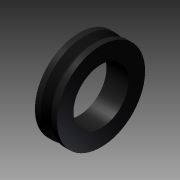
# Autodesk Inventor part: 8 ball cable roller
Saved by Autodesk Inventor 2012 (Build 160160000, 160)
## iProperties
Created: 2013-12-03
Part Number: 8 ball cable roller
Material: Default
Document SubType Name: Modeling
Designer: Bryce
Density: 1 g/cm^3
Author: Bryce
Autodesk Inventor part; units mm, degrees
ref_plane "YZ Plane" through (0, 0, 0) normal (1, 0, 0) x (0, 1, 0)
ref_plane "XZ Plane" through (0, 0, 0) normal (0, 1, 0) x (-1, 0, 0)
ref_plane "XY Plane" through (0, 0, 0) normal (0, 0, 1) x (1, 0, 0)
sketch "Sketch1" plane through (0, 0, 0) normal (0, 0, 1) x (1, 0, 0)
  line L0 (0, 0) -> (9.525, 0) construction
  line L1 (1.5875, 7.9375) -> (7.9375, 7.9375)
  line L2 (7.9375, 7.9375) -> (7.9375, 12.7)
  line L3 (1.5875, 12.7) -> (1.5875, 7.9375)
  line L4 (3.175, 12.7) -> (4.7625, 11.1125)
  line L5 (4.7625, 11.1125) -> (6.35, 12.7)
  line L6 (7.9375, 12.7) -> (6.35, 12.7)
  line L7 (3.175, 12.7) -> (1.5875, 12.7)
  line L8 (1.5875, 7.9375) -> (0, 7.9375)
  line L9 (0, 7.9375) -> (0, 6.6675)
  line L10 (0, 6.6675) -> (0.635, 6.6675)
  line L11 (0.635, 6.6675) -> (0.635, 5.08)
  line L12 (0.635, 5.08) -> (0, 5.08)
  line L13 (0, 5.08) -> (0, 2.54)
  line L14 (0, 2.54) -> (9.525, 2.54)
  line L15 (9.525, 2.54) -> (9.525, 5.08)
  line L16 (9.525, 5.08) -> (8.89, 5.08)
  line L17 (8.89, 5.08) -> (8.89, 6.6675)
  line L18 (8.89, 6.6675) -> (9.525, 6.6675)
  line L19 (9.525, 6.6675) -> (9.525, 7.9375)
  line L20 (9.525, 7.9375) -> (7.9375, 7.9375)
  point P0 (4.7625, 7.9375)
  dimension "d0" = 6.35
  dimension "d1" = 4.7625
  dimension "d2" = 1.5875
  dimension "d3" = 7.9375
  dimension "d5" = 11.1125
  dimension "d6" = 9.525
  dimension "d7" = 1.27
  dimension "d8" = 1.5875
  dimension "d9" = 2.54
  dimension "d10" = 0.635
  constraints: 42 end point, 13 parallel, 10 collinear, 3 perpendicular, 2 horizontal, 2 vertical alignment, 1 midpoint
  measures "d0" distance of L1.start L1.end
  measures "d1" distance of L3.start L1.start
  measures "d2" distance from line of L0.start L3
  measures "d3" distance between parallel lines of L0 L1
  measures "d5" distance from line of L0 L4.end
  measures "d6" distance of L13.end L14.end
  measures "d7" distance of L8.end L9.end
  measures "d8" distance of L10.end L11.end
  measures "d9" distance between parallel lines of L0 L14
  measures "d10" distance of L9.end L10.end
revolve "Revolution1" add sketch "Sketch1" angle 360 about axis through (0, 0, 0) along (1, 0, 0) contours L3 L7 L4 L5 L6 L2 L1
body "Solid1"
